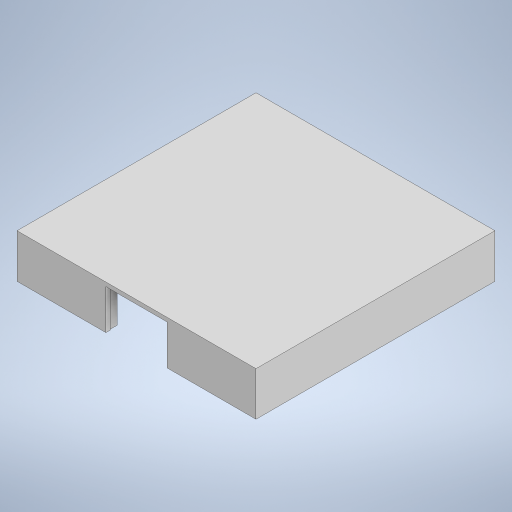
# Autodesk Inventor part: keypad cover good
Saved by Autodesk Inventor 2023 (Build 270158000, 158)
## iProperties
Created: 2023-01-16
Part Number: keypad cover good
Material: Generic
Document SubType Name: Modeling
Designer: appab
Density: 1 g/cm^3
Appearance: Default
Author: appab
Autodesk Inventor part; units mm, degrees
ref_plane "YZ Plane" through (0, 0, 0) normal (1, 0, 0) x (0, 1, 0)
ref_plane "XZ Plane" through (0, 0, 0) normal (0, 1, 0) x (-1, 0, 0)
ref_plane "XY Plane" through (0, 0, 0) normal (0, 0, 1) x (1, 0, 0)
sketch "Sketch1" plane through (0, 0, 0) normal (0, 1, 0) x (-1, 0, 0)
  line L0 (0, 0) -> (-76.2, 0)
  line L1 (-76.2, 0) -> (-76.2, -76.2)
  line L2 (-76.2, -76.2) -> (0, -76.2)
  line L3 (0, -76.2) -> (0, 0)
  line L4 (-8.89, -8.89) -> (-67.31, -8.89)
  line L5 (-67.31, -8.89) -> (-67.31, -67.31)
  line L6 (-67.31, -67.31) -> (-8.89, -67.31)
  line L7 (-8.89, -67.31) -> (-8.89, -8.89)
  line L8 (-8.89, -8.89) -> (-67.31, -67.31) construction
  line L9 (-67.31, -8.89) -> (-8.89, -67.31) construction
  point P0 (-38.1, -38.1)
  dimension "d0" = 76.2
  dimension "d1" = 76.2
  dimension "d2" = 58.42
  dimension "d3" = 58.42
  constraints: 20 end point, 4 parallel, 2 horizontal, 2 midpoint, 2 perpendicular
  measures "d0" distance of L2.end L1.end
  measures "d1" distance of L1.end L0.end
  measures "d2" distance of L6.end L5.end
  measures "d3" distance of L5.end L4.end
extrude "Extrusion1" add sketch "Sketch1" along normal blind 12.7
sketch "Sketch2" plane through (0, 12.7, 0) normal (0, 1, 0) x (1, 0, 0)
  line L0 (0, 76.2) -> (0, 0) projected
  line L1 (76.2, 0) -> (76.2, 76.2) projected
  line L2 (0, 0) -> (76.2, 0)
  line L3 (76.2, 0) -> (76.2, 76.2)
  line L4 (76.2, 76.2) -> (0, 76.2)
  line L5 (0, 76.2) -> (0, 0)
  constraints: 8 end point, 2 parallel, 1 horizontal, 1 perpendicular
extrude "Extrusion2" add sketch "Sketch2" along normal blind 1.27
sketch "Sketch3" plane through (0, 0, 0) normal (0, -1, 0) x (1, 0, 0)
  line L0 (67.31, -67.31) -> (67.31, -8.89) construction
  line L1 (76.2, 0) -> (76.2, -76.2) construction
  line L2 (67.31, -8.89) -> (76.2, 0) construction
  line L3 (67.31, -67.31) -> (76.2, -76.2) construction
  line L4 (8.89, -67.31) -> (0, -76.2) construction
  line L5 (8.89, -8.89) -> (8.89, -67.31) construction
  line L6 (8.89, -8.89) -> (0, 0) construction
  circle A0 centre (71.755, -4.445) radius 1.7399
  circle A1 centre (71.755, -71.755) radius 1.7399
  circle A2 centre (4.445, -4.445) radius 1.7399
  circle A3 centre (4.445, -71.755) radius 1.7399
  dimension "d8" = 3.4798
  dimension "d9" = 3.4798
  dimension "d10" = 3.4798
  dimension "d11" = 3.4798
  constraints: 8 end point, 4 centre point, 4 midpoint, 1 perpendicular
  measures "d8" diameter of A0
  measures "d9" diameter of A1
  measures "d10" diameter of A2
  measures "d11" diameter of A3
extrude "Extrusion3" cut sketch "Sketch3" against normal blind 12.7
sketch "Sketch4" plane through (0, 0, 0) normal (0, -1, 0) x (1, 0, 0)
  line L0 (67.31, -67.31) -> (67.31, -8.89) projected
  line L1 (67.31, -8.89) -> (72.39, -8.89)
  line L2 (72.39, -8.89) -> (72.39, -67.31)
  line L3 (72.39, -67.31) -> (67.31, -67.31)
  line L4 (67.31, -67.31) -> (67.31, -8.89)
  circle A0 centre (38.1, -38.1) radius 2.0553 construction
  line L5 (8.89, -3.81) -> (67.31, -3.81)
  line L6 (8.89, -8.89) -> (8.89, -3.81)
  line L7 (67.31, -8.89) -> (8.89, -8.89)
  line L8 (67.31, -3.81) -> (67.31, -8.89)
  line L9 (3.81, -67.31) -> (3.81, -8.89)
  line L10 (8.89, -67.31) -> (3.81, -67.31)
  line L11 (8.89, -8.89) -> (8.89, -67.31)
  line L12 (3.81, -8.89) -> (8.89, -8.89)
  line L13 (67.31, -72.39) -> (8.89, -72.39)
  line L14 (67.31, -67.31) -> (67.31, -72.39)
  line L15 (8.89, -67.31) -> (67.31, -67.31)
  line L16 (8.89, -72.39) -> (8.89, -67.31)
  point P0 (0, 0)
  dimension "d14" = 5.08
  dimension "d17" = 360
  constraints: 32 end point, 2 parallel, 1 centre point, 1 horizontal, 1 perpendicular, 37 other
  measures "d14" distance of L2.end L3.end
extrude "Extrusion4" cut sketch "Sketch4" against normal blind 12.7 contours L0 L1 L2 L3 | L14 L13 L16 L15 | L7 L6 L5 L8 | L10 L9 L12 L11
sketch "Sketch5" plane through (0, 0, 0) normal (0, -1, 0) x (1, 0, 0)
  line L0 (0, 0) -> (76.2, 0) projected
  line L1 (47.85, 0) -> (28.35, 0)
  line L2 (28.35, 0) -> (28.35, -1.5)
  line L3 (28.35, -1.5) -> (38.1, -1.5)
  line L4 (47.85, -1.5) -> (47.85, 0)
  line L5 (8.89, -3.81) -> (67.31, -3.81) construction
  line L6 (38.1, -3.81) -> (38.1, 0) construction
  line L7 (48.1, -3.81) -> (28.1, -3.81)
  line L8 (28.1, -3.81) -> (28.1, -1.5)
  line L9 (48.1, -1.5) -> (48.1, -3.81)
  line L10 (28.1, -1.5) -> (38.1, -1.5)
  line L11 (47.85, -1.5) -> (48.1, -1.5)
  point P0 (28.35, 0)
  dimension "d21" = 19.5
  dimension "d22" = 1.5
  dimension "d23" = 20
  constraints: 20 end point, 5 parallel, 4 point on line, 3 perpendicular, 2 horizontal, 2 midpoint, 2 other
  measures "d21" distance of L4.start L2.end
  measures "d22" distance of L2.end L1.end
  measures "d23" distance of L8.end L9.start
extrude "Extrusion5" cut sketch "Sketch5" against normal blind 12.7
sketch "Sketch6" plane through (0, 0, 0) normal (0, -1, 0) x (1, 0, 0)
  line L0 (0, -76.2) -> (0, 0) projected
  line L1 (0, -33.85) -> (1, -33.85)
  line L2 (1, -33.85) -> (1, -42.35)
  line L3 (1, -42.35) -> (0, -42.35)
  line L4 (0, -42.35) -> (0, -33.85)
  line L5 (3.81, -67.31) -> (3.81, -8.89) construction
  line L6 (3.81, -38.1) -> (0, -38.1) construction
  line L7 (3.81, -29.35) -> (1, -29.35)
  line L8 (1, -29.35) -> (1, -46.85)
  line L9 (1, -46.85) -> (3.81, -46.85)
  line L10 (3.81, -46.85) -> (3.81, -29.35)
  dimension "d26" = 1
  dimension "d27" = 8.5
  dimension "d28" = 17.5
  constraints: 18 end point, 4 parallel, 3 horizontal, 2 midpoint, 2 perpendicular, 2 point on line, 2 other
  measures "d26" distance of L2.end L3.end
  measures "d27" distance of L1.end L2.end
  measures "d28" distance of L8.end L7.end
extrude "Extrusion6" cut sketch "Sketch6" against normal blind 4
sketch "Sketch7" plane through (0, 4, 0) normal (0, -1, 0) x (1, 0, 0)
  line L0 (1, -33.85) -> (1, -29.35) projected
  line L1 (0, -76.2) -> (0, -42.35) projected
  line L2 (1, -33.85) -> (0, -33.85)
  line L3 (0, -33.85) -> (0, -42.35)
  line L4 (0, -42.35) -> (1, -42.35)
  line L5 (1, -42.35) -> (1, -33.85)
  point P0 (0, 0)
  constraints: 8 end point, 2 parallel, 1 horizontal, 1 perpendicular
extrude "Extrusion7" add sketch "Sketch7" along normal blind 1.5
body "Solid1"
